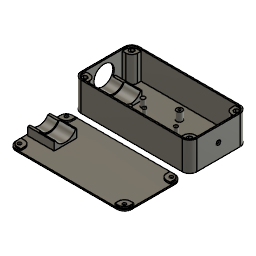
AC Box v1 (Autodesk Fusion 360 design; units mm, degrees)
Autodesk Fusion 360 part; units mm, degrees
sketch "Sketch1" plane through (0, 0, 0) normal (0, 1, 0) x (1, 0, 0)
  line L0 (12.7, -25.4) -> (-165.1, -25.4)
  line L1 (-177.8, -12.7) -> (-177.8, 63.5)
  line L2 (-165.1, 76.2) -> (12.7, 76.2)
  line L3 (25.4, 63.5) -> (25.4, -12.7)
  arc A0 (-165.1, 76.2) -> (-177.8, 63.5) centre (-165.1, 63.5) ccw
  arc A1 (-177.8, -12.7) -> (-165.1, -25.4) centre (-165.1, -12.7) ccw
  arc A2 (25.4, 63.5) -> (12.7, 76.2) centre (12.7, 63.5) ccw
  arc A3 (12.7, -25.4) -> (25.4, -12.7) centre (12.7, -12.7) ccw
  line L4 (-158.75, 57.15) -> (-177.8, 57.15)
  line L5 (-177.8, 57.15) -> (-177.8, 76.2)
  line L6 (-177.8, 76.2) -> (-158.75, 76.2)
  line L7 (-158.75, 76.2) -> (-158.75, 57.15)
  line L8 (-164.275, 68.9844) -> (-168.275, 71.2938)
  line L9 (-168.275, 71.2938) -> (-172.275, 68.9844)
  line L10 (-172.275, 68.9844) -> (-172.275, 64.3656)
  line L11 (-172.275, 64.3656) -> (-168.275, 62.0562)
  line L12 (-168.275, 62.0562) -> (-164.275, 64.3656)
  line L13 (-164.275, 64.3656) -> (-164.275, 68.9844)
  line L14 (6.35, 76.2) -> (25.4, 76.2)
  line L15 (25.4, 57.15) -> (6.35, 57.15)
  line L16 (11.875, 68.9844) -> (11.875, 64.3656)
  line L17 (19.875, 64.3656) -> (19.875, 68.9844)
  line L18 (25.4, 76.2) -> (25.4, 57.15)
  line L19 (19.875, 68.9844) -> (15.875, 71.2938)
  line L20 (15.875, 71.2938) -> (11.875, 68.9844)
  line L21 (11.875, 64.3656) -> (15.875, 62.0562)
  line L22 (15.875, 62.0562) -> (19.875, 64.3656)
  line L23 (6.35, 57.15) -> (6.35, 76.2)
  line L24 (-177.8, -6.35) -> (-158.75, -6.35)
  line L25 (-158.75, -25.4) -> (-177.8, -25.4)
  line L26 (-172.275, -13.5656) -> (-172.275, -18.1844)
  line L27 (-164.275, -18.1844) -> (-164.275, -13.5656)
  line L28 (-158.75, -6.35) -> (-158.75, -25.4)
  line L29 (-164.275, -13.5656) -> (-168.275, -11.2562)
  line L30 (-168.275, -11.2562) -> (-172.275, -13.5656)
  line L31 (-172.275, -18.1844) -> (-168.275, -20.4938)
  line L32 (-168.275, -20.4938) -> (-164.275, -18.1844)
  line L33 (-177.8, -25.4) -> (-177.8, -6.35)
  line L34 (6.35, -6.35) -> (25.4, -6.35)
  line L35 (25.4, -25.4) -> (6.35, -25.4)
  line L36 (11.875, -13.5656) -> (11.875, -18.1844)
  line L37 (19.875, -18.1844) -> (19.875, -13.5656)
  line L38 (25.4, -6.35) -> (25.4, -25.4)
  line L39 (19.875, -13.5656) -> (15.875, -11.2562)
  line L40 (15.875, -11.2562) -> (11.875, -13.5656)
  line L41 (11.875, -18.1844) -> (15.875, -20.4938)
  line L42 (15.875, -20.4938) -> (19.875, -18.1844)
  line L43 (6.35, -25.4) -> (6.35, -6.35)
  circle A4 centre (-168.275, 66.675) radius 3.175
  circle A5 centre (-168.275, -15.875) radius 3.175
  circle A6 centre (15.875, -15.875) radius 3.175
  circle A7 centre (15.875, 66.675) radius 3.175
  point P0 (0, -25.4)
  point P1 (-177.8, -25.4)
  point P2 (25.4, 76.2)
  point P3 (-168.275, 66.675)
  point P4 (-6.35, 76.2)
  point P5 (-19.05, 63.5)
  point P6 (-6.35, 63.5)
  point P7 (15.875, 66.675)
  point P8 (-165.1, -6.35)
  point P9 (-177.8, -19.05)
  point P10 (-165.1, -19.05)
  point P11 (-168.275, -15.875)
  point P12 (-6.35, -6.35)
  point P13 (-19.05, -19.05)
  point P14 (-6.35, -19.05)
  point P15 (15.875, -15.875)
  dimension "d1" = 177.8
  dimension "d3" = 12.7
  dimension "d4" = 12.7
  dimension "d5" = 12.7
  dimension "d6" = 12.7
  dimension "d7" = 4
  dimension "d12" = 6.35
  dimension "d13" = 6.35
  dimension "d14" = 6.35
  dimension "d15" = 6.35
  dimension "d138" = 203.2
  constraint vertical L1
  constraint horizontal L2
  constraint vertical L3
  constraint tangent L1 A0
  constraint tangent L2 A0
  constraint coincident P1 L1
  constraint coincident P1 L0
  constraint tangent L1 A1
  constraint tangent L0 A1
  constraint coincident P2 L2
  constraint coincident P2 L3
  constraint tangent L2 A2
  constraint tangent L3 A2
  constraint tangent L3 A3
  constraint tangent L0 A3
  constraint horizontal L4
  constraint vertical L5
  constraint horizontal L6
  constraint vertical L7
  constraint coincident P3 A4.centre
  constraint coincident P11 A5.centre
  constraint coincident P15 A6.centre
  constraint coincident P7 A7.centre
  measures "d1" distance of P0 L25.end
  measures "d3" radius of A0
  measures "d4" radius of A1
  measures "d5" radius of A2
  measures "d6" radius of A3
  measures "d7" distance of P3 L13
  measures "d12" diameter of A4
  measures "d13" diameter of A5
  measures "d14" diameter of A6
  measures "d15" diameter of A7
  measures "d138" distance of L1 L3
  measures "d149" distance of L27.end
  measures "d150" distance of L27.end
  measures "d152" distance of L27.end
  measures "d153" distance of L27.end
extrude "Extrude1" add sketch "Sketch1" along normal blind 50.8 contours L0 L3 A3 L34 L35 L38 L43 | L0 L1 L2 L3 L4 L7 L15 L23 L24 L28 L34 L43 | L0 L1 A1 L24 L25 L28 L33 | L2 L3 A2 L14 L15 L18 L23 | L1 L2 A0 L4 L5 L6 L7 | L8 L9 L10 L11 L12 L13 | L16 L17 L19 L20 L21 L22 | L26 L27 L29 L30 L31 L32 | L36 L37 L39 L40 L41 L42 | A4 | A5 | A6 | A7 makes body 1
shell "Shell1" thickness 2.54 removed faces 1 at (-48.6833, 50.8, -8.4667) on bodies 1
extrude "Extrude2" add sketch "Sketch1" along normal blind 48.26 contours L0 L3 A3 L34 L35 L38 L43 | L0 L1 A1 L24 L25 L28 L33 | L2 L3 A2 L14 L15 L18 L23 | L1 L2 A0 L4 L5 L6 L7 bodies 1
extrude "Extrude3" add sketch "Sketch1" along normal blind 43.18 contours L8 L9 L10 L11 L12 L13 | L16 L17 L19 L20 L21 L22 | L26 L27 L29 L30 L31 L32 | L36 L37 L39 L40 L41 L42 bodies 1
fillet "Fillet1" radius 10.16 4 edges at (-158.75, 25.4, -57.15) (-158.75, 25.4, 6.35) (6.35, 25.4, -57.15) (6.35, 25.4, 6.35) on bodies 1
sketch "Sketch3" plane through (0, 0, 0) normal (0, 1, 0) x (1, 0, 0)
  line L0 (-165.1, -50.8) -> (12.7, -50.8)
  line L1 (25.4, -63.5) -> (25.4, -139.7)
  line L2 (12.7, -152.4) -> (-165.1, -152.4)
  line L3 (-177.8, -139.7) -> (-177.8, -63.5)
  arc A0 (-165.1, -50.8) -> (-177.8, -63.5) centre (-165.1, -63.5) ccw
  arc A1 (25.4, -63.5) -> (12.7, -50.8) centre (12.7, -63.5) ccw
  arc A2 (-177.8, -139.7) -> (-165.1, -152.4) centre (-165.1, -139.7) ccw
  arc A3 (12.7, -152.4) -> (25.4, -139.7) centre (12.7, -139.7) ccw
  line L4 (-168.91, -69.85) -> (-177.8, -69.85)
  line L5 (-177.8, -69.85) -> (-177.8, -50.8)
  line L6 (-177.8, -50.8) -> (-158.75, -50.8)
  line L7 (-158.75, -50.8) -> (-158.75, -59.69)
  circle A4 centre (-168.275, -60.325) radius 3
  line L8 (25.4, -133.35) -> (16.51, -133.35)
  line L9 (6.35, -143.51) -> (6.35, -152.4)
  line L10 (6.35, -152.4) -> (25.4, -152.4)
  line L11 (25.4, -152.4) -> (25.4, -133.35)
  circle A5 centre (15.875, -142.875) radius 3
  circle A6 centre (15.875, -60.325) radius 3
  circle A7 centre (-168.275, -142.875) radius 3
  line L12 (-177.8, -152.4) -> (-158.75, -152.4)
  line L13 (-158.75, -152.4) -> (-158.75, -143.51)
  line L14 (-168.91, -133.35) -> (-177.8, -133.35)
  line L15 (-177.8, -133.35) -> (-177.8, -152.4)
  line L16 (16.51, -69.85) -> (25.4, -69.85)
  line L17 (25.4, -69.85) -> (25.4, -50.8)
  line L18 (25.4, -50.8) -> (6.35, -50.8)
  line L19 (6.35, -50.8) -> (6.35, -59.69)
  arc A8 (-168.91, -69.85) -> (-158.75, -59.69) centre (-168.91, -59.69) ccw
  arc A9 (-158.75, -143.51) -> (-168.91, -133.35) centre (-168.91, -143.51) ccw
  arc A10 (6.35, -59.69) -> (16.51, -69.85) centre (16.51, -59.69) ccw
  arc A11 (16.51, -133.35) -> (6.35, -143.51) centre (16.51, -143.51) ccw
  arc A12 (-165.1, -53.34) -> (-175.26, -63.5) centre (-165.1, -63.5) ccw
  line L20 (-175.26, -139.7) -> (-175.26, -63.5)
  arc A13 (-175.26, -139.7) -> (-165.1, -149.86) centre (-165.1, -139.7) ccw
  line L21 (12.7, -149.86) -> (-165.1, -149.86)
  arc A14 (12.7, -149.86) -> (22.86, -139.7) centre (12.7, -139.7) ccw
  line L22 (22.86, -63.5) -> (22.86, -139.7)
  arc A15 (22.86, -63.5) -> (12.7, -53.34) centre (12.7, -63.5) ccw
  line L23 (-165.1, -53.34) -> (12.7, -53.34)
  line L24 (6.35, -53.34) -> (3.81, -53.34)
  circle A16 centre (-168.275, -60.325) radius 5
  circle A17 centre (-168.275, -142.875) radius 5
  circle A18 centre (15.875, -142.875) radius 5
  circle A19 centre (15.875, -60.325) radius 5
  dimension "d28" = 12.7
  dimension "d29" = 12.7
  dimension "d30" = 12.7
  dimension "d31" = 12.7
  dimension "d32" = 6
  dimension "d34" = 6
  dimension "d35" = 6
  dimension "d36" = 6
  dimension "d39" = 19.05
  dimension "d40" = 10.16
  dimension "d41" = 10.16
  dimension "d42" = 10.16
  dimension "d43" = 10.16
  dimension "d44" = 2.54
  dimension "d68" = 10
  dimension "d69" = 10
  dimension "d70" = 10
  dimension "d71" = 10
  dimension "d139" = 198.12
  constraint horizontal L0
  constraint vertical L1
  constraint horizontal L2
  constraint vertical L3
  constraint tangent L0 A0
  constraint tangent L3 A0
  constraint tangent L0 A1
  constraint tangent L1 A1
  constraint tangent L3 A2
  constraint tangent L2 A2
  constraint tangent L1 A3
  constraint tangent L2 A3
  constraint horizontal L4
  constraint vertical L5
  constraint horizontal L6
  constraint vertical L7
  constraint horizontal L8
  constraint vertical L9
  constraint horizontal L10
  constraint vertical L11
  constraint horizontal L12
  constraint vertical L13
  constraint horizontal L14
  constraint vertical L15
  constraint horizontal L16
  constraint vertical L17
  constraint horizontal L18
  constraint vertical L19
  constraint tangent L4 A8
  constraint tangent L7 A8
  constraint tangent L13 A9
  constraint tangent L14 A9
  constraint tangent L16 A10
  constraint tangent L19 A10
  constraint tangent L8 A11
  constraint tangent L9 A11
  constraint horizontal L24
  constraint coincident L23 L24.start
  constraint coincident L19 L24.start
  constraint concentric A4 A16
  constraint concentric A7 A17
  constraint concentric A5 A18
  constraint concentric A6 A19
  measures "d28" radius of A0
  measures "d29" radius of A1
  measures "d30" radius of A2
  measures "d31" radius of A3
  measures "d32" diameter of A4
  measures "d34" diameter of A5
  measures "d35" diameter of A6
  measures "d36" diameter of A7
  measures "d39" distance of L12.start L14.end
  measures "d40" radius of A8
  measures "d41" radius of A9
  measures "d42" radius of A10
  measures "d43" radius of A11
  measures "d68" diameter of A16
  measures "d69" diameter of A17
  measures "d70" diameter of A18
  measures "d71" diameter of A19
  measures "d139" distance of L20 L22
extrude "Extrude5" add sketch "Sketch3" along normal blind 2.54 separate body contours L0 L3 A0 L4 L5 L6 L7 A12 L20 L23 | L0 L7 L19 L23 L24 | L0 L1 A1 L16 L17 L18 L19 L22 A15 L23 | L4 L7 L8 L9 L13 L14 L16 L19 A8 A9 A10 A11 L20 L21 L22 L23 L24 | L4 L7 A8 A12 L20 L23 | L3 L4 L14 L20 | L16 L19 A10 L22 A15 L23 | L2 L3 A2 L12 L13 L14 L15 L20 A13 L21 | L13 L14 A9 L20 A13 L21 | L1 L8 L16 L22 | L1 L2 A3 L8 L9 L10 L11 L21 A14 L22 | L2 L9 L13 L21 | L8 L9 A11 L21 A14 L22 | A16 | A17 | A18 | A19 makes body 2
extrude "Extrude6" add sketch "Sketch3" along normal blind 5.08 contours L4 L7 A8 A12 L20 L23 | L16 L19 A10 L22 A15 L23 | L13 L14 A9 L20 A13 L21 | L8 L9 A11 L21 A14 L22 | A16 | A17 | A18 | A19 bodies 2
extrude "Extrude8" cut sketch "Sketch3" along normal blind 2 contours A16 | A17 | A18 | A19 bodies 2
sketch "Sketch5" plane through (-175.26, 0, 0) normal (1, 0, 0) x (0, 0, -1)
  line L0 (57.15, 2.54) -> (57.15, 48.26)
  line L1 (57.15, 48.26) -> (63.5, 48.26)
  line L2 (63.5, 48.26) -> (63.5, 50.8)
  line L3 (63.5, 50.8) -> (-12.7, 50.8)
  line L4 (-12.7, 50.8) -> (-12.7, 48.26)
  line L5 (-12.7, 48.26) -> (-6.35, 48.26)
  line L6 (-6.35, 48.26) -> (-6.35, 2.54)
  line L7 (-6.35, 2.54) -> (57.15, 2.54)
  line L8 (-6.35, 2.54) -> (57.15, 2.54) construction
  line L9 (25.4, 2.54) -> (25.4, 50.8) construction
  circle A0 centre (25.4, 26.67) radius 17.75
  circle A1 centre (25.4, 26.67) radius 19.7546
  line L10 (4.0115, 26.67) -> (46.7885, 26.67) construction
  line L11 (43.15, 26.67) -> (43.15, 2.54)
  line L12 (7.65, 26.67) -> (7.65, 2.54)
  line L13 (5.6454, 26.67) -> (5.6454, 2.54)
  line L14 (45.1546, 26.67) -> (45.1546, 2.54)
  line L15 (5.6454, 2.54) -> (5.6454, 17.78) construction
  line L16 (5.6454, 17.78) -> (45.1546, 17.78)
  circle A2 centre (-101.6, 25.6641) radius 17.75
  line L17 (-83.85, 25.6655) -> (-83.8482, 2.54)
  line L18 (-81.8454, 25.6641) -> (-81.8454, 2.54)
  circle A3 centre (-101.6, 25.6641) radius 19.7546
  line L19 (-121.3546, 17.78) -> (-81.8454, 17.78)
  line L20 (-119.35, 25.6648) -> (-119.3509, 2.54)
  line L21 (-121.3546, 2.54) -> (-121.3546, 17.78) construction
  line L22 (-121.3546, 25.6641) -> (-121.3546, 2.54)
  line L23 (-25.4, 0) -> (-50.8, 0) construction
  line L24 (-50.8, 0) -> (-152.4, 0) construction
  line L25 (-101.6, 0) -> (-101.6, 54.6365) construction
  line L26 (25.4, 46.4246) -> (-149.722, 46.4246) construction
  line L27 (25.4, 50.8) -> (-152.4, 50.8) construction
  line L28 (-121.3546, 2.54) -> (-81.8454, 2.54)
  line L29 (25.4, 6.9154) -> (25.4, 15.4154)
  line L30 (-101.6, 5.9095) -> (-101.6, 14.4095)
  point P0 (25.4, 26.67)
  dimension "d78" = 35.5
  dimension "d88" = 39.5092
  dimension "d90" = 15.24
  dimension "d95" = 35.5
  dimension "d96" = 39.5092
  dimension "d97" = 15.24
  dimension "d120" = 8.5
  dimension "d121" = 8.5
  constraint coincident L6.end L7.start
  constraint coincident L0.start L7.end
  constraint midpoint L8 L9.start
  constraint midpoint L3 L9.end
  constraint midpoint L9 P0
  constraint concentric A0 A1
  constraint midpoint L10 P0
  constraint coincident P0 A0.centre
  constraint perpendicular L9 L10
  constraint coincident A0 L11.start
  constraint coincident L10 L11.start
  constraint coincident L8 L11.end
  constraint tangent A0 L11
  constraint coincident L10 L12.start
  constraint coincident A0 L12.start
  constraint coincident L8 L12.end
  constraint tangent A0 L12
  constraint coincident A1 L13.start
  constraint coincident L10 L13.start
  constraint coincident L8 L13.end
  constraint tangent A1 L13
  constraint coincident A1 L14.start
  constraint coincident L10 L14.start
  constraint coincident L8 L14.end
  constraint tangent A1 L14
  constraint coincident L13 L15.end
  constraint coincident L14 L16.end
  constraint perpendicular L14 L16
  constraint concentric A2 A3
  constraint coincident L17.start A2
  constraint tangent A2 L17
  constraint coincident L20.start A2
  constraint tangent A2 L20
  constraint coincident L22.start A3
  constraint tangent A3 L22
  constraint coincident L18.start A3
  constraint tangent L18 A3
  constraint coincident L19.start L22
  constraint coincident L19.end L18
  constraint perpendicular L18 L19
  constraint perpendicular L22 L23
  constraint perpendicular L22 L24
  constraint midpoint L24 L25.start
  constraint perpendicular L24 L25
  constraint coincident A1 L26.start
  constraint coincident L9 L26.start
  constraint tangent A1 L26
  constraint perpendicular L25 L27
  constraint horizontal L28
  constraint coincident A1 L29.start
  constraint coincident L9 L29.start
  constraint perpendicular L16 L29
  constraint coincident A3 L30.start
  constraint coincident L25 L30.start
  constraint parallel L25 L30
  measures "d78" diameter of A0
  measures "d88" diameter of A1
  measures "d90" distance of L13.end L15.end
  measures "d95" diameter of A2
  measures "d96" diameter of A3
  measures "d97" distance of L19.start L21.start
  measures "d120" distance of L29.start L29.end
  measures "d121" distance of L30.start L30.end
extrude "Extrude10" cut sketch "Sketch5" against normal blind 7.62 contours A0 L16 | A0 L16 bodies 1
sketch "Sketch6" plane through (0, 50.8, 0) normal (0, 1, 0) x (-1, 0, 0)
  line L0 (-22.86, -63.5) -> (-22.86, 12.7)
  arc A0 (-12.7, 22.86) -> (-22.86, 12.7) centre (-12.7, 12.7) ccw
  line L1 (-12.7, 22.86) -> (165.1, 22.86)
  arc A1 (175.26, 12.7) -> (165.1, 22.86) centre (165.1, 12.7) ccw
  line L2 (175.26, 12.7) -> (175.26, -63.5)
  arc A2 (165.1, -73.66) -> (175.26, -63.5) centre (165.1, -63.5) ccw
  line L3 (165.1, -73.66) -> (-12.7, -73.66)
  arc A3 (-22.86, -63.5) -> (-12.7, -73.66) centre (-12.7, -63.5) ccw
  arc A4 (-25.4, -63.5) -> (-12.7, -76.2) centre (-12.7, -63.5) ccw
  line L4 (-12.7, -76.2) -> (165.1, -76.2)
  arc A5 (165.1, -76.2) -> (177.8, -63.5) centre (165.1, -63.5) ccw
  line L5 (177.8, -63.5) -> (177.8, -57.15)
  line L6 (177.8, -57.15) -> (177.8, 6.35)
  arc A6 (177.8, 12.7) -> (165.1, 25.4) centre (165.1, 12.7) ccw
  line L7 (165.1, 25.4) -> (-12.7, 25.4)
  arc A7 (-12.7, 25.4) -> (-25.4, 12.7) centre (-12.7, 12.7) ccw
  line L8 (-25.4, 12.7) -> (-25.4, 6.35)
  line L9 (-25.4, 6.35) -> (-25.4, -57.15)
  line L10 (177.8, -25.4) -> (181.8, -25.4) construction
  line L11 (181.8, -25.4) -> (111.8, -25.4) construction
  line L12 (181.8001, -43.15) -> (181.8001, -7.65) construction
  line L13 (181.8001, -43.15) -> (181.8001, -7.65) construction
  line L14 (181.8001, -7.65) -> (157.8001, -7.65) construction
  line L15 (157.8001, -7.65) -> (157.8001, -43.15) construction
  line L16 (157.8001, -43.15) -> (181.8001, -43.15) construction
  line L17 (157.8001, -5.9) -> (157.8001, -44.9)
  line L18 (157.8001, -44.9) -> (112.0801, -44.9)
  line L19 (112.0801, -44.9) -> (112.0801, -5.9)
  line L20 (112.0801, -5.9) -> (157.8001, -5.9)
  line L21 (157.8001, -43.15) -> (181.8001, -43.15)
  line L22 (181.8001, -43.15) -> (181.8001, -7.65)
  line L23 (181.8001, -7.65) -> (157.8001, -7.65)
  line L24 (157.8001, -7.65) -> (157.8001, -43.15)
  line L25 (157.8001, -25.4) -> (128.8001, -25.4) construction
  line L26 (128.8001, -44.9) -> (128.8001, -5.9)
  line L27 (112.0801, -5.9) -> (114.6201, -5.9) construction
  line L28 (114.6201, -5.9) -> (114.6201, -44.9) construction
  line L29 (114.6201, -44.9) -> (112.0801, -44.9) construction
  line L30 (112.0801, -44.9) -> (112.0801, -5.9) construction
  line L31 (118.8201, -41.4) -> (118.8201, -9.4) construction
  line L32 (114.6201, -11.0399) -> (123.0201, -11.0399) construction
  line L33 (114.6201, -11.0399) -> (118.8201, -11.0399)
  line L34 (118.8201, -9.4) -> (118.8201, -13.6) construction
  circle A8 centre (118.8201, -13.6) radius 4.2 construction
  line L35 (118.8201, -25.4) -> (118.8201, -37.211) construction
  circle A9 centre (118.8201, -37.211) radius 4.2 construction
  line L36 (120.1628, -32.65) -> (120.1628, -18.15) construction
  line L37 (120.65, -41.4) -> (120.65, -9.4) construction
  circle A10 centre (118.8201, -13.6) radius 3.7
  circle A11 centre (118.8201, -37.211) radius 3.7
  line L38 (177.8, 6.35) -> (177.8, 12.7)
  line L39 (-25.4, -57.15) -> (-25.4, -63.5)
  point P0 (157.8001, -25.4)
  point P1 (118.8201, -25.4)
  point P2 (120.1628, -25.4)
  point P3 (120.65, -25.4)
  dimension "d81" = 4
  dimension "d82" = 70
  dimension "d84" = 35.5
  dimension "d85" = 24
  dimension "d86" = 39
  dimension "d87" = 45.72
  dimension "d89" = 29
  dimension "d102" = 2.54
  dimension "d103" = 32
  dimension "d105" = 8.4
  dimension "d106" = 24
  dimension "d107" = 4.0001
  dimension "d108" = 4.2
  dimension "d109" = 19.5
  dimension "d110" = 4.2
  dimension "d111" = 4.2
  dimension "d112" = 11.811
  dimension "d113" = 8.4
  dimension "d114" = 14.5
  dimension "d115" = 32
  dimension "d116" = 7.4
  dimension "d117" = 7.4
  constraint perpendicular L5 L10
  constraint perpendicular L5 L11
  constraint perpendicular L10 L12
  constraint perpendicular L13 L14
  constraint parallel L13 L15
  constraint parallel L14 L16
  constraint coincident L15 P0
  constraint perpendicular L17 L18
  constraint parallel L17 L19
  constraint parallel L18 L20
  constraint horizontal L21
  constraint horizontal L23
  constraint vertical L24
  constraint coincident P0 L25.start
  constraint perpendicular L15 L25
  constraint midpoint L25.end L26
  constraint coincident L20 L26.end
  constraint perpendicular L20 L26
  constraint horizontal L27
  constraint vertical L28
  constraint horizontal L29
  constraint vertical L30
  constraint coincident L18 L28.end
  constraint midpoint L31 P1
  constraint coincident L11 P1
  constraint perpendicular L11 L31
  constraint coincident L28 L32.start
  constraint perpendicular L28 L32
  constraint midpoint L32 L33.end
  constraint coincident L31 L34.end
  constraint coincident L34.end A8.centre
  constraint tangent L28 A8
  constraint coincident P1 L35.start
  constraint coincident L31 L35.end
  constraint coincident L35.end A9.centre
  constraint midpoint L36 P2
  constraint coincident L11 P2
  constraint perpendicular L11 L36
  constraint midpoint L37 P3
  constraint coincident L11 P3
  constraint perpendicular L32 L37
  constraint concentric A9 A11
  measures "d81" distance of L10.start L10.end
  measures "d82" distance of L10.end L11.end
  measures "d84" distance of L12.start L12.end
  measures "d85" distance of L12.start L15.end
  measures "d86" distance of L17.end L17.start
  measures "d87" distance of L17.start L19.end
  measures "d89" distance of P0 L25.end
  measures "d102" distance of L19.end L27.end
  measures "d103" distance of L31.start L31.end
  measures "d105" distance of L32.start L32.end
  measures "d106" distance of L12 L17
  measures "d107" distance of L6 L12
  measures "d108" distance of L32.start L33.end
  measures "d109" distance of L11 L20
  measures "d110" distance of L28 L31
  measures "d111" distance of L31.end L34.end
  measures "d112" distance of P1 L35.end
  measures "d113" diameter of A9
  measures "d114" distance of L36.start L36.end
  measures "d115" distance of L37.start L37.end
  measures "d116" diameter of A10
  measures "d117" diameter of A11
extrude "Extrude11" add sketch "Sketch5" along normal blind 46.4566 contours L7 L11 L14 L16 | L7 A1 L11 L12 L16 | L7 L12 L13 L16 bodies 1
extrude "Extrude12" add sketch "Sketch5" along normal blind 18.0086 contours A0 A1 L16 L29 | A0 A1 L16 L29 bodies 1
extrude "Extrude13" add sketch "Sketch5" along normal blind 46.4566 contours L17 L18 A3 L19 L28 | L17 A3 L20 L28 | A3 L19 L20 L22 L28 bodies 2
extrude "Extrude14" add sketch "Sketch5" along normal blind 18.0086 contours A2 L17 A3 L19 L30 | L17 A3 L19 | A2 A3 L19 L20 L30 | A3 L19 L20 bodies 2
extrude "Extrude15" add sketch "Sketch6" against normal blind 48.26 contours A10 | A11 bodies 1
extrude "Extrude16" cut 2 faces at (-118.5457, 50.8, -12.3976) (-118.5457, 50.8, -36.0086) along direction (0, -1, 0) blind 35.3822 on bodies 1 bodies 1
sketch "Sketch7" plane through (0, 17.78, 0) normal (0, 1, 0) x (-1, 0, 0)
  line L0 (175.26, 117.5029) -> (175.26, 121.3546)
  line L1 (175.26, 121.3546) -> (128.8034, 121.3546)
  line L2 (128.8034, 121.3546) -> (128.8034, 119.7131)
  line L3 (128.8034, 119.7131) -> (157.2514, 119.7131)
  line L4 (157.2514, 119.7131) -> (157.2514, 117.5029)
  line L5 (157.2514, 117.5029) -> (175.26, 117.5029)
  line L6 (124.46, 129.54) -> (193.04, 129.54)
  line L7 (193.04, 129.54) -> (193.04, 76.2)
  line L8 (193.04, 76.2) -> (124.46, 76.2)
  line L9 (124.46, 76.2) -> (124.46, 129.54)
  constraint horizontal L6
  constraint vertical L7
  constraint horizontal L8
  constraint vertical L9
extrude "Extrude17" cut sketch "Sketch7" against normal blind 1 contours L0 L1 L2 L3 L4 L5 | L6 L7 L8 L9 bodies 2
sketch "Sketch8" plane through (0, 50.8, 0) normal (0, 1, 0) x (-1, 0, 0)
  arc A0 (175.26, 12.7) -> (165.1, 22.86) centre (165.1, 12.7) ccw
  line L0 (175.26, 12.7) -> (175.26, -63.5)
  arc A1 (165.1, -73.66) -> (175.26, -63.5) centre (165.1, -63.5) ccw
  line L1 (165.1, -73.66) -> (-12.7, -73.66)
  arc A2 (-22.86, -63.5) -> (-12.7, -73.66) centre (-12.7, -63.5) ccw
  arc A3 (-25.4, -63.5) -> (-12.7, -76.2) centre (-12.7, -63.5) ccw
  line L2 (-12.7, -76.2) -> (165.1, -76.2)
  arc A4 (165.1, -76.2) -> (177.8, -63.5) centre (165.1, -63.5) ccw
  line L3 (177.8, -63.5) -> (177.8, -57.15)
  line L4 (177.8, -57.15) -> (177.8, 6.35)
  arc A5 (177.8, 12.7) -> (165.1, 25.4) centre (165.1, 12.7) ccw
  line L5 (-25.4, 6.35) -> (-25.4, -57.15)
  line L6 (42.44, 17.2622) -> (102.14, 17.2622)
  line L7 (102.14, 17.2622) -> (102.14, -22.6378)
  line L8 (102.14, -22.6378) -> (42.44, -22.6378)
  line L9 (42.44, -22.6378) -> (42.44, 17.2622)
  line L10 (-3.56, 10.8122) -> (42.44, 10.8122)
  line L11 (42.44, 10.8122) -> (42.44, -16.1878)
  line L12 (42.44, -16.1878) -> (-3.56, -16.1878)
  line L13 (-3.56, -16.1878) -> (-3.56, 10.8122)
  line L14 (177.8, 6.35) -> (177.8, 12.7)
  line L15 (-25.4, -57.15) -> (-25.4, -63.5)
  line L16 (0.04, -31.04) -> (66.04, -31.04)
  line L17 (66.04, -31.04) -> (66.04, -66.04)
  line L18 (66.04, -66.04) -> (0.04, -66.04)
  line L19 (0.04, -66.04) -> (0.04, -31.04)
  line L20 (102.14, 17.2622) -> (102.6558, 17.2622) construction
  line L21 (102.6558, 17.2622) -> (102.6558, 16.2622) construction
  line L22 (102.6558, 16.2622) -> (102.14, 16.2622) construction
  line L23 (102.14, 16.2622) -> (102.14, 17.2622) construction
  line L24 (102.14, 17.2622) -> (101.14, 17.2622) construction
  line L25 (101.14, 17.2622) -> (101.14, -96.481) construction
  line L26 (101.14, -96.481) -> (102.14, -96.481) construction
  line L27 (102.14, -96.481) -> (102.14, 17.2622) construction
  line L28 (101.14, 17.2622) -> (101.14, 15.2622) construction
  line L29 (101.14, 15.2622) -> (100.14, 15.2622) construction
  circle A6 centre (100.14, 15.2622) radius 1 construction
  circle A7 centre (100.14, 15.2622) radius 1
  line L30 (102.14, -22.6378) -> (100.14, -22.6378)
  line L31 (100.14, -22.6378) -> (100.14, -20.6378) construction
  line L32 (100.14, -20.6378) -> (102.14, -20.6378) construction
  line L33 (102.14, -20.6378) -> (102.14, -22.6378)
  circle A8 centre (100.14, -20.6378) radius 1
  line L34 (42.44, -22.6378) -> (44.44, -22.6378) construction
  line L35 (44.44, -22.6378) -> (44.44, -20.6378) construction
  line L36 (44.44, -20.6378) -> (42.44, -20.6378) construction
  line L37 (42.44, -20.6378) -> (42.44, -22.6378) construction
  circle A9 centre (44.44, -20.6378) radius 1
  line L38 (42.44, 17.2622) -> (44.44, 17.2622) construction
  line L39 (44.44, 17.2622) -> (44.44, 15.2622) construction
  line L40 (44.44, 15.2622) -> (42.44, 15.2622) construction
  line L41 (42.44, 15.2622) -> (42.44, 17.2622) construction
  circle A10 centre (44.44, 15.2622) radius 1
  circle A11 centre (44.44, 15.2622) radius 3.175
  circle A12 centre (100.14, 15.2622) radius 3.175
  circle A13 centre (100.14, -20.6378) radius 3.175
  circle A14 centre (44.44, -20.6378) radius 3.175
  line L42 (63.7527, -66.04) -> (2.3527, -66.04)
  line L43 (2.3527, -66.04) -> (2.3527, -31.04) construction
  line L44 (63.7527, -66.04) -> (63.7527, -31.04) construction
  line L45 (2.3527, -51.54) -> (2.3527, -45.54) construction
  line L46 (2.3527, -51.54) -> (2.3527, -45.54) construction
  line L47 (0.04, -45.1876) -> (0.04, -51.8924) construction
  line L48 (0.04, -51.8924) -> (2.3527, -51.54) construction
  line L49 (2.3527, -51.54) -> (2.3527, -45.54)
  line L50 (2.3527, -45.54) -> (0.04, -45.54)
  line L51 (0.04, -45.54) -> (0.04, -51.54)
  line L52 (0.04, -51.54) -> (2.3527, -51.54)
  line L53 (2.3527, -45.54) -> (66.037, -45.54) construction
  line L54 (66.037, -45.54) -> (66.04, -51.54) construction
  line L55 (66.04, -51.54) -> (2.3527, -51.54) construction
  line L56 (63.7527, -45.54) -> (66.04, -45.54)
  line L57 (66.04, -45.54) -> (66.04, -51.54)
  line L58 (66.04, -51.54) -> (63.7527, -51.54)
  line L59 (63.7527, -51.54) -> (63.7527, -45.54)
  line L60 (63.7527, -48.54) -> (66.2527, -48.54) construction
  circle A15 centre (66.2527, -48.54) radius 2
  circle A16 centre (66.2527, -48.54) radius 5.08
  line L61 (2.3527, -48.54) -> (-0.1473, -48.54) construction
  circle A17 centre (-0.1473, -48.54) radius 2
  circle A18 centre (-0.1473, -48.54) radius 5.08
  circle A19 centre (44.44, -20.6378) radius 0.5
  circle A20 centre (44.44, 15.2622) radius 0.5
  circle A21 centre (100.14, 15.2622) radius 0.5
  circle A22 centre (100.14, -20.6378) radius 0.5
  point P0 (33.0527, -66.04)
  point P1 (2.3527, -48.54)
  dimension "d134" = 59.7
  dimension "d135" = 39.9
  dimension "d136" = 46
  dimension "d137" = 27
  dimension "d140" = 66
  dimension "d141" = 35
  dimension "d142" = 1
  dimension "d143" = 1
  dimension "d144" = 2
  dimension "d145" = 1
  dimension "d146" = 2
  dimension "d147" = 2
  dimension "d148" = 2
  dimension "d149" = 2
  dimension "d150" = 2
  dimension "d151" = 2
  dimension "d152" = 2
  dimension "d153" = 2
  dimension "d154" = 2
  dimension "d155" = 6.35
  dimension "d156" = 6.35
  dimension "d157" = 6.35
  dimension "d158" = 6.35
  dimension "d159" = 61.4
  dimension "d160" = 6
  dimension "d161" = 2.3127
  dimension "d162" = 2.5
  dimension "d163" = 4
  dimension "d164" = 10.16
  dimension "d165" = 2.5
  dimension "d166" = 4
  dimension "d167" = 10.16
  dimension "d168" = 1
  dimension "d169" = 1
  dimension "d170" = 1
  dimension "d171" = 1
  constraint horizontal L6
  constraint vertical L7
  constraint horizontal L8
  constraint vertical L9
  constraint horizontal L10
  constraint vertical L11
  constraint horizontal L12
  constraint vertical L13
  constraint midpoint L9 L11
  constraint horizontal L16
  constraint vertical L17
  constraint horizontal L18
  constraint vertical L19
  constraint horizontal L20
  constraint vertical L21
  constraint horizontal L22
  constraint vertical L23
  constraint horizontal L24
  constraint vertical L25
  constraint horizontal L26
  constraint vertical L27
  constraint coincident L25 L28.end
  constraint perpendicular L25 L29
  constraint coincident L29.end A6.centre
  constraint tangent L22 A6
  constraint concentric A6 A7
  constraint horizontal L30
  constraint vertical L31
  constraint horizontal L32
  constraint vertical L33
  constraint coincident L31.end L32.start
  constraint horizontal L34
  constraint vertical L35
  constraint horizontal L36
  constraint vertical L37
  constraint coincident L35.end L36.start
  constraint horizontal L38
  constraint vertical L39
  constraint horizontal L40
  constraint vertical L41
  constraint coincident L39.end L40.start
  constraint concentric A10 A11
  constraint concentric A7 A12
  constraint concentric A8 A13
  constraint concentric A9 A14
  constraint midpoint L42 P0
  constraint coincident L18 P0
  constraint coincident L18 L42.end
  constraint coincident L16 L43.end
  constraint perpendicular L16 L43
  constraint coincident L16 L44.end
  constraint perpendicular L16 L44
  constraint midpoint L45 P1
  constraint coincident L43 P1
  constraint parallel L43 L45
  constraint parallel L46 L47
  constraint perpendicular L49 L50
  constraint parallel L49 L51
  constraint parallel L50 L52
  constraint parallel L53 L55
  constraint horizontal L56
  constraint vertical L57
  constraint horizontal L58
  constraint vertical L59
  constraint coincident L44 L56.start
  constraint coincident L53 L56.start
  constraint midpoint L19 L47
  constraint midpoint L19 L51
  constraint midpoint L17 L57
  constraint midpoint L59 L60.start
  constraint perpendicular L17 L60
  constraint coincident L60.end A15.centre
  constraint concentric A15 A16
  constraint coincident P1 L61.start
  constraint perpendicular L19 L61
  constraint coincident L61.end A17.centre
  constraint concentric A17 A18
  constraint concentric A9 A19
  constraint concentric A11 A20
  constraint concentric A8 A22
  measures "d134" distance of L6.start L6.end
  measures "d135" distance of L6.start L8.end
  measures "d136" distance of L10.start L10.end
  measures "d137" distance of L10.start L12.end
  measures "d140" distance of L16.start L16.end
  measures "d141" distance of L16.start L18.end
  measures "d142" distance of L6.end L22.end
  measures "d143" distance of L6.end L24.end
  measures "d144" distance of L24.end L28.end
  measures "d145" distance of L28.end L29.end
  measures "d146" distance of L7.end L30.end
  measures "d147" distance of L7.end L32.end
  measures "d148" diameter of A8
  measures "d149" distance of L8.end L34.end
  measures "d150" distance of L8.end L36.end
  measures "d151" diameter of A9
  measures "d152" distance of L6.start L38.end
  measures "d153" distance of L6.start L40.end
  measures "d154" diameter of A10
  measures "d155" diameter of A11
  measures "d156" diameter of A12
  measures "d157" diameter of A13
  measures "d158" diameter of A14
  measures "d159" distance of L42.start L42.end
  measures "d160" distance of L45.start L45.end
  measures "d161" distance of L45.end L50.end
  measures "d162" distance of L60.start L60.end
  measures "d163" diameter of A15
  measures "d164" diameter of A16
  measures "d165" distance of P1 L61.end
  measures "d166" diameter of A17
  measures "d167" diameter of A18
  measures "d168" diameter of A19
  measures "d169" diameter of A20
  measures "d170" diameter of A21
  measures "d171" diameter of A22
extrude "Extrude18" add sketch "Sketch8" against normal blind 48.26 contours L6 L9 A11 | L6 L9 A11 | L6 L7 A12 | L6 L7 A12 | L7 L8 L30 L33 A13 | L7 L8 L30 L33 A13 | L8 L9 A14 | L8 L9 A14 | L19 L49 L50 L52 A18 | L19 L51 A17 A18 | L17 L57 A15 A16 | L17 L56 L58 L59 A16 | L19 L49 L50 L51 L52 A17 | L17 L56 L57 L58 L59 A15 | A7 | A8 | A9 | A10 bodies 1
extrude "Extrude19" cut 6 faces at (-46.7115, 50.8, 15.42) (-46.7115, 50.8, -20.48) (-70.2871, 50.8, -48.2876) (-101.1392, 50.8, -22.6838) (-99.7883, 50.8, 17.5119) (-3.8796, 50.8, -48.1883) along direction (0, -1, 0) blind 33.02 on bodies 1 bodies 1
sketch "Sketch9" plane through (22.86, 0, 0) normal (-1, 0, 0) x (0, 0, 1)
  line L0 (-63.5, 48.26) -> (-57.15, 48.26)
  line L1 (-57.15, 48.26) -> (-57.15, 2.54)
  line L2 (-57.15, 2.54) -> (6.35, 2.54)
  line L3 (6.35, 2.54) -> (6.35, 48.26)
  line L4 (6.35, 48.26) -> (12.7, 48.26)
  line L5 (12.7, 48.26) -> (12.7, 50.8)
  line L6 (12.7, 50.8) -> (-63.5, 50.8)
  line L7 (-63.5, 50.8) -> (-63.5, 48.26)
  line L8 (6.35, 25.4) -> (-57.15, 25.4) construction
  line L9 (-25.4, 0) -> (-25.4, 50.8) construction
  circle A0 centre (-25.4, 25.4) radius 3.81
  point P0 (-25.4, 25.4)
  dimension "d176" = 7.62
  constraint midpoint L3 L8.start
  constraint midpoint L1 L8.end
  constraint midpoint L9 P0
  constraint coincident L8 P0
  constraint coincident L6 L9.end
  constraint coincident P0 A0.centre
  measures "d176" diameter of A0
extrude "Extrude20" cut sketch "Sketch9" against normal blind 5.08 contours A0 bodies 1
move_body "Move1" bodies 2 to x (1, 0, 0) y (0, 1, 0) z (0, 0, 1) at (0, 0, -12.7)
equation "d88 = 1.398 in + 4 mm"
equation "d96 = 1.398 in + 4 mm"
